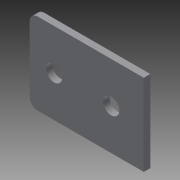
# Autodesk Inventor part: Pneumatic Spring attach Point
Saved by Autodesk Inventor 2015 (Build 190159000, 159)
## iProperties
Created: 2015-01-25
Part Number: Pneumatic Spring attach Point
Material: Generic
Document SubType Name: Modeling
Designer: chapale16
Density: 1 g/cm^3
Appearance: Default
Author: chapale16
Autodesk Inventor part; units mm, degrees
ref_plane "YZ Plane" through (0, 0, 0) normal (1, 0, 0) x (0, 1, 0)
ref_plane "XZ Plane" through (0, 0, 0) normal (0, 1, 0) x (-1, 0, 0)
ref_plane "XY Plane" through (0, 0, 0) normal (0, 0, 1) x (1, 0, 0)
sketch "Sketch1" plane through (0, 0, 0) normal (0, 0, 1) x (1, 0, 0)
  line L0 (0, 0) -> (19.05, 0)
  line L1 (19.05, 0) -> (19.05, -31.75)
  line L2 (19.05, -31.75) -> (0, -31.75)
  line L3 (0, -31.75) -> (0, 0)
  circle A0 centre (9.525, -15.875) radius 3.175
  line L4 (19.05, -31.75) -> (44.45, -31.75)
  line L5 (44.45, -31.75) -> (44.45, 0)
  line L6 (44.45, 0) -> (19.05, 0)
  line L7 (19.05, 0) -> (19.05, -31.75)
  circle A1 centre (31.75, -15.875) radius 3.175
  dimension "d0" = 19.05
  dimension "d1" = 31.75
  dimension "d2" = 6.35
  dimension "d5" = 25.4
  constraints: 16 end point, 4 parallel, 2 centre point, 2 horizontal, 2 perpendicular
  measures "d0" distance of L1.end L2.end
  measures "d1" distance of L0.end L1.end
  measures "d2" diameter of A0
  measures "d5" distance of L6.end L5.end
extrude "Extrusion1" add sketch "Sketch1" along normal blind 2.54 contours L0 L1 L2 L3
extrude "Extrusion2" cut sketch "Sketch1" along normal blind 2.54 contours L6 L5 L4 L1
extrude "Extrusion3" add sketch "Sketch1" along normal blind 2.54 contours L6 L5 L4 L1
fillet "Fillet1" radius 3.175 1 edges at (0, 0, 1.27)
fillet "Fillet2" radius 3.175 1 edges at (0, -31.75, 1.27)
body "Solid1"
